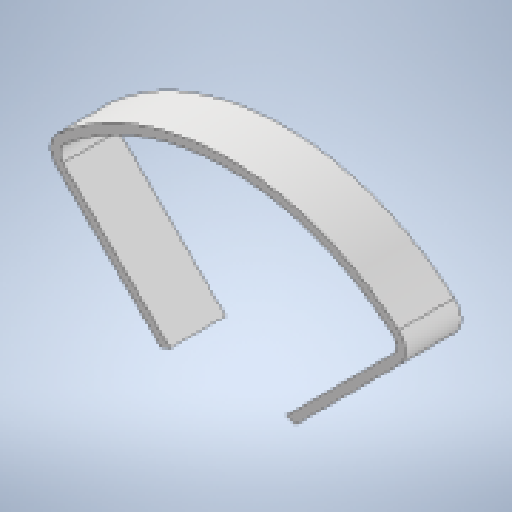
# Autodesk Inventor part: Tolva_Salida
Saved by Autodesk Inventor 2024 (Build 280153000, 153)
## iProperties
Created: 2024-07-17
Part Number: Tolva_Salida
Material: Genérico
Document SubType Name: Modeling
Designer: sergi
Density: 1 g/cm^3
Appearance: Valor por defecto
Author: sergi
Autodesk Inventor part; units mm, degrees
ref_plane "YZ Plane" through (0, 0, 0) normal (1, 0, 0) x (0, 1, 0)
sketch "Boceto1" plane through (0, 0, 0) normal (0, 0, 1) x (1, 0, 0)
  circle A0 centre (-50, -88) radius 1.5 projected
  circle A1 centre (50, -88) radius 1.5 projected
  circle A2 centre (88, -50) radius 1.5 projected
  circle A3 centre (88, 50) radius 1.5 projected
  circle A4 centre (50, 88) radius 1.5 projected
  circle A5 centre (-50, 88) radius 1.5 projected
  circle A6 centre (-88, 50) radius 1.5 projected
  circle A7 centre (-88, -50) radius 1.5 projected
  arc A8 (29.6244, 31.0386) -> (29.5223, 33.9623) centre (28.2102, 32.4528) ccw projected
  line L0 (29.6244, 31.0386) -> (9.8759, 11.2901) projected
  line L1 (-9.8759, 11.2901) -> (-29.6244, 31.0386) projected
  arc A9 (-29.5223, 33.9623) -> (-29.6244, 31.0386) centre (-28.2102, 32.4528) ccw projected
  arc A10 (29.5223, 33.9623) -> (-29.5223, 33.9623) centre (0, 0) ccw projected
  line L2 (100, -100) -> (100, 100) projected
  line L3 (100, 100) -> (-100, 100) projected
  line L4 (-100, 100) -> (-100, -100) projected
  line L5 (-100, -100) -> (100, -100) projected
  line L6 (10.7339, 9.8854) -> (30.7558, 29.9072)
  arc A11 (30.7558, 29.9072) -> (30.572, 35.1698) centre (28.2102, 32.4528) ccw
  arc A12 (30.572, 35.1698) -> (-30.572, 35.1698) centre (0, 0) ccw
  arc A13 (-30.572, 35.1698) -> (-30.7558, 29.9072) centre (-28.2102, 32.4528) ccw
  line L7 (-30.7558, 29.9072) -> (-12.0679, 11.2194)
  line L8 (31.8102, 5.2085) -> (31.8102, 100)
  line L9 (30.2102, 29.3617) -> (30.2102, 100)
  line L10 (-31.8102, 32.4528) -> (-31.8102, 100)
  line L11 (-30.2102, 31.7383) -> (-30.2102, 100)
  circle A14 centre (55, 0) radius 2.5 projected
  arc A15 (-5.2203, -12.3413) -> (5.2203, -12.3413) centre (0, 0) ccw projected
  arc A16 (54.4847, -4.9734) -> (5.2203, -12.3413) centre (44.1778, -104.4408) ccw projected
  arc A17 (54.4847, -4.9734) -> (54.4847, 4.9734) centre (55, 0) ccw projected
  arc A18 (11.6313, 9.8854) -> (54.4847, 4.9734) centre (44.1778, 104.4408) ccw projected
  arc A19 (-54.4847, 4.9734) -> (-11.6313, 9.8854) centre (-44.1778, 104.4408) ccw projected
  arc A20 (-54.4847, 4.9734) -> (-54.4847, -4.9734) centre (-55, 0) ccw projected
  arc A21 (-5.2203, -12.3413) -> (-54.4847, -4.9734) centre (-44.1778, -104.4408) ccw projected
  circle A22 centre (0, 0) radius 4 projected
  circle A23 centre (-55, 0) radius 2.5 projected
  arc A24 (9.8759, 11.2901) -> (-9.8759, 11.2901) centre (0, 0) ccw
  line L12 (-30.7558, 29.9072) -> (-10.7339, 9.8854)
  arc A25 (5.2203, 12.3413) -> (-5.2203, 12.3413) centre (0, 0) ccw
  line L13 (10.9657, 10.1171) -> (30.7558, 29.9072)
  arc A26 (30.7558, 29.9072) -> (30.572, 35.1698) centre (28.2102, 32.4528) ccw
  arc A27 (30.572, 35.1698) -> (-30.572, 35.1698) centre (0, 0) ccw
  arc A28 (-30.572, 35.1698) -> (-30.7558, 29.9072) centre (-28.2102, 32.4528) ccw
  line L14 (11.6313, 9.8854) -> (-11.6313, 9.8854) projected
  line L15 (9.8759, 11.2901) -> (-9.8759, 11.2901)
  point P0 (-30.2102, 32.4528)
  point P1 (30.2102, 32.4528)
  point P2 (31.8102, 32.4528)
  point P3 (-30.2102, 35.4811)
  point P4 (31.8102, 32.4528)
  point P5 (30.2102, 35.4811)
  point P6 (44.1778, 104.4408)
  point P7 (-44.1778, 104.4408)
  dimension "d0" = 1.6
  constraints: 20 point on circle, 18 end point, 8 centre point, 7 point on line, 4 tangent, 2 parallel, 2 perpendicular, 1 horizontal, 8 other
  measures "d0" distance between parallel lines of L0 L6
ref_plane "Plano de trabajo1" through (-60, -15, 10) normal (0, 0, 1) x (1, 0, 0)
ref_plane "Plano de trabajo3" through (-60, -13.4, 10) normal (0, 0, 1) x (1, 0, 0)
extrude "Extrusión1" add sketch "Boceto1" along normal up to surface (10 mm away) contours A8 L9 L6 L14 L12 L7 A13 A12 L11 A9 L1 L15 L0 | L9 A12 A11 L6 | L9 L3 L8 A11 A12 | A12 A13 L10 L3 L11
ref_plane "Plano de trabajo5" through (0, 32.4528, 0) normal (-1, 0, 0) x (0, 0, 1)
sketch "Boceto4" plane through (0, 32.4528, 0) normal (-1, 0, 0) x (0, 0, 1)
  line L0 (10, -1.4142) -> (10, -21.1627) projected
  line L1 (10, 0) -> (10, -1.4142) projected
  line L2 (10, 67.5472) -> (10, 0) projected
  line L3 (10, 0) -> (10, 67.5472) projected
  line L4 (10, -2.5456) -> (10, 0) projected
  line L5 (10, -22.5674) -> (10, -2.5456) projected
  line L6 (10, -2.5456) -> (10, -22.5674) projected
  line L7 (10, 0) -> (10, -2.5456) projected
  line L8 (10, 67.5472) -> (10, 0) projected
  line L9 (10, 0) -> (10, 67.5472) projected
  line L10 (10, -1.4142) -> (10, 0) projected
  line L11 (10, -21.1627) -> (10, -1.4142) projected
  line L12 (-103, 70.5472) -> (-78, 70.5472) projected
  line L13 (-78, 70.5472) -> (-53, 70.5472) projected
  line L14 (-53, 70.5472) -> (-28, 70.5472) projected
  line L15 (-28, 70.5472) -> (-3, 70.5472) projected
  line L16 (-3, 70.5472) -> (22, 70.5472) projected
  line L17 (22, 70.5472) -> (47, 70.5472) projected
  line L18 (47, 70.5472) -> (72, 70.5472) projected
  line L19 (72, 70.5472) -> (97, 70.5472) projected
  line L20 (97, 70.5472) -> (122, 70.5472) projected
  line L21 (122, 70.5472) -> (147, 70.5472) projected
  line L22 (10, -22.5674) -> (63.7597, 70.5472)
  line L23 (10, -22.5674) -> (117.5195, -22.5674) construction
  point P0 (0, -32.4528)
  dimension "d9" = 60
  constraints: 4 end point, 1 equal length, 1 horizontal, 1 point on line
  measures "d9" angle of L23 L22
sketch "Boceto5" plane through (-10.7339, 9.8854, 10) normal (0, 0, 1) x (1, 0, 0)
  line L0 (-18.8905, 21.1532) -> (0.858, 1.4047) projected
  arc A0 (-19.4762, 22.5674) -> (-18.8905, 21.1532) centre (-17.4762, 22.5674) ccw projected
  line L1 (-19.4762, 90.1146) -> (-19.4762, 22.5674) projected
  line L2 (-21.0762, 90.1146) -> (-19.4762, 90.1146) projected
  line L3 (-21.0762, 22.5674) -> (-21.0762, 90.1146) projected
  arc A1 (-21.0762, 22.5674) -> (-20.0218, 20.0218) centre (-17.4762, 22.5674) ccw projected
  line L4 (0, 0) -> (-20.0218, 20.0218) projected
  line L5 (21.4679, 0) -> (0, 0) projected
  line L6 (41.4897, 20.0218) -> (21.4679, 0) projected
  arc A2 (41.4897, 20.0218) -> (42.5441, 22.5674) centre (38.9441, 22.5674) ccw projected
  line L7 (42.5441, 90.1146) -> (42.5441, 22.5674) projected
  line L8 (40.9441, 90.1146) -> (42.5441, 90.1146) projected
  line L9 (40.9441, 22.5674) -> (40.9441, 90.1146) projected
  arc A3 (40.3583, 21.1532) -> (40.9441, 22.5674) centre (38.9441, 22.5674) ccw projected
  line L10 (20.6098, 1.4047) -> (40.3583, 21.1532) projected
  line L11 (0.858, 1.4047) -> (20.6098, 1.4047) projected
  point P0 (10.7339, -9.8854)
sweep "Barrido2" add profiles "Boceto5" path "Boceto4" path curves L22
ref_plane "Plano de trabajo6" through (-31.8102, 100, 0) normal (0, 1, 0) x (1, 0, 0)
split "Dividir2" plane through (-31.8102, 100, 0) removes the side toward (0, 1, 0)
